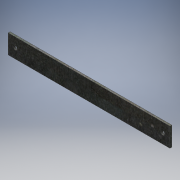
# Autodesk Inventor part: ballastBar
Saved by Autodesk Inventor 2016 (Build 200138000, 138)
## iProperties
Created: 2015-12-25
Part Number: ballastBar
Material: Steel
Document SubType Name: Modeling
Designer: Artur
Density: 7.85 g/cm^3
Appearance: Plate
Mass: 52.6714 g
Surface Area: 75.16 cm^2
Volume: 6.70973 cm^3
Author: Artur
Autodesk Inventor part; units mm, degrees
ref_plane "YZ Plane" through (0, 0, 0) normal (1, 0, 0) x (0, 1, 0)
ref_plane "XZ Plane" through (0, 0, 0) normal (0, 1, 0) x (-1, 0, 0)
ref_plane "XY Plane" through (0, 0, 0) normal (0, 0, 1) x (1, 0, 0)
sketch "Sketch1" plane through (0, 0, 0) normal (0, 1, 0) x (-1, 0, 0)
  line L0 (0, 0) -> (169, 0)
  line L1 (169, 0) -> (169, -20)
  line L2 (169, -20) -> (0, -20)
  line L3 (0, -20) -> (0, 0)
  dimension "d0" = 169
  dimension "d1" = 20
  constraints: 8 end point, 2 parallel, 1 horizontal, 1 perpendicular
  measures "d0" distance of L0.start L0.end
  measures "d1" distance of L0.end L1.end
extrude "Extrusion1" add sketch "Sketch1" along normal blind 2
sketch "Sketch2" plane through (0, 0, 0) normal (0, -1, 0) x (1, 0, 0)
  line L0 (0, 0) -> (0, -20) projected
  line L1 (0, -10) -> (-169, -10) construction
  line L2 (-169, -20) -> (-169, 0) projected
  line L3 (-84.5, -10) -> (-84.5, 52.7002) construction
  point P0 (-161.5, -10)
  point P1 (-7.5, -10)
  dimension "d6" = 154
  constraints: 4 end point, 3 midpoint, 1 point on line, 1 symmetric about line, 1 vertical
  measures "d6" diameter of point (-161.5, -10) L3
hole "Hole1" at (-161.5, 0, -10) at (-7.5, 0, -10) direction (0, 1, 0) diameter 4 end through all
sketch "Sketch3" plane through (0, 0, 0) normal (0, -1, 0) x (1, 0, 0)
  line L0 (-169, -20) -> (-169, 0) construction
  line L1 (-169, -10) -> (0, -10) construction
  line L2 (0, 0) -> (0, -20) construction
  line L3 (-169, 0.75) -> (0, 0.75)
  line L4 (-169, 0.75) -> (-169, -10)
  line L5 (0, 0.75) -> (0, -10)
  line L6 (-169, -20.75) -> (0, -20.75)
  line L7 (-169, -20.75) -> (-169, -10)
  line L8 (0, -20.75) -> (0, -10)
  dimension "d15" = 21.5
  constraints: 14 end point, 2 collinear, 2 midpoint, 2 point on line, 2 symmetric about line, 1 perpendicular
  measures "d15" diameter of L3 L1
extrude "Extrusion2" cut sketch "Sketch3" against normal blind 10 keep common part
body "Solid1"
